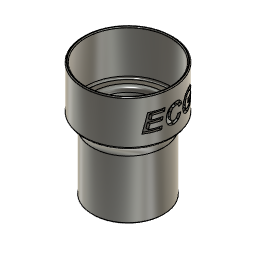
v1.0.0-ecg-fydro-flask (Autodesk Fusion 360 design; units mm, degrees)
Autodesk Fusion 360 part; units mm, degrees
sketch "Sketch1" plane through (0, 0, 0) normal (0, 0, 1) x (1, 0, 0)
  circle A0 centre (-30, 35) radius 40
  dimension "d6" = 80
  measures "d6" diameter of A0
extrude "Extrude1" add sketch "Sketch1" along normal blind 80
sketch "Sketch2" plane through (0, 0, 80) normal (0, 0, 1) x (-1, 0, 0)
  circle A0 centre (30, -35) radius 40
  circle A1 centre (30, -35) radius 35
  dimension "d3" = 70
  constraint concentric A0 A1
  measures "d3" diameter of A1
extrude "Extrude2" cut sketch "Sketch2" against normal blind 70 contours A1
sketch "Sketch3" plane through (0, 0, 80) normal (0, 0, 1) x (-1, 0, 0)
  circle A0 centre (30, -35) radius 35
  circle A1 centre (30, -35) radius 40
  circle A2 centre (30, -35) radius 50
  dimension "d9" = 100
  constraint concentric A0 A2
  measures "d9" diameter of A2
extrude "Extrude3" add sketch "Sketch3" along normal blind 50 contours A1 | A2
fillet "Fillet1" radius 15 1 edges at (-67.2931, 20.5354, 80)
sketch "Sketch6" plane through (0, 0, 130) normal (0, 0, 1) x (-1, 0, 0)
  circle A0 centre (30, -35) radius 35
  circle A1 centre (30, -35) radius 50
  circle A2 centre (30, -35) radius 47.5
  dimension "d15" = 95
  constraint concentric A0 A2
  measures "d15" diameter of A2
extrude "Extrude5" cut sketch "Sketch6" against normal blind 50 contours A2
fillet "Fillet2" radius 5 1 edges at (2.6315, 47.6565, 80)
fillet "Fillet3" radius 1 2 edges at (16.6164, 53.0808, 130) (14.2855, 17.8233, 130)
fillet "Fillet4" radius 1 1 edges at (-67.2931, 20.5354, 0)
sketch "Sketch7" plane through (0, 0, 0) normal (1, 0, 0) x (0, 1, 0)
  line L0 (6.9052, 86.7655) -> (69.3523, 86.7655) construction
  line L1 (69.3523, 86.7655) -> (69.3523, 120.0906) construction
  line L2 (69.3523, 120.0906) -> (6.9052, 120.0906) construction
  line L3 (6.9052, 120.0906) -> (6.9052, 86.7655) construction
  dimension "d24" = 20
  text T0 "ECG" font "Arial" height 20 bold italic align centre middle in box 62.4471 x 33.3251 at (6.9052, 86.7655) x (1, 0) y (0, 1) spacing 1
extrude "Extrude6" cut sketch "Sketch7" along normal blind 20 text T0
fillet "Fillet5" radius 2 1 edges at (16.6164, 53.0808, 80)
fillet "Fillet6" radius 2 1 edges at (14.2855, 17.8233, 80)
fillet "Fillet7" radius 2 1 edges at (2.6315, 22.3435, 10)
